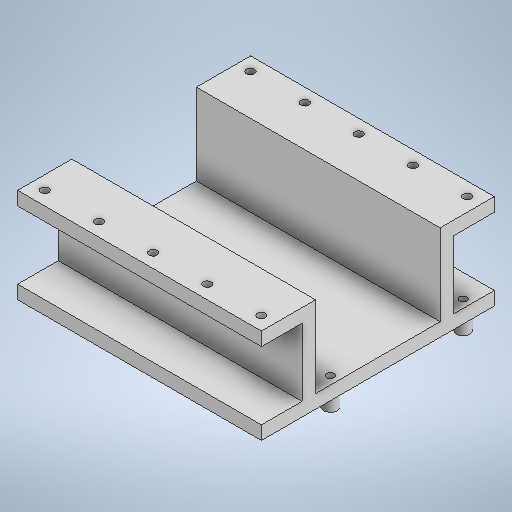
# Autodesk Inventor part: Battery_zig
Saved by Autodesk Inventor 2025 (Build 290162010, 162A)
## iProperties
Created: 2024-09-12
Part Number: Battery_zig
Material: Generic
Document SubType Name: Modeling
Designer: fist5
Density: 1 g/cm^3
Appearance: Default
Author: fist5
Autodesk Inventor part; units mm, degrees
ref_plane "YZ Plane" through (0, 0, 0) normal (1, 0, 0) x (0, 1, 0)
ref_plane "XZ Plane" through (0, 0, 0) normal (0, 1, 0) x (-1, 0, 0)
ref_plane "XY Plane" through (0, 0, 0) normal (0, 0, 1) x (1, 0, 0)
sketch "Sketch1" plane through (0, 0, 0) normal (0, 1, 0) x (-1, 0, 0)
  line L0 (45, -43) -> (-45, -43)
  line L1 (-45, -43) -> (-45, 43)
  line L2 (-45, 43) -> (45, 43)
  line L3 (45, 43) -> (45, -43)
  line L4 (45, -43) -> (-45, 43) construction
  line L5 (-45, -43) -> (45, 43) construction
  point P0 (0, 0)
  dimension "d0" = 90
  dimension "d1" = 86
  constraints: 12 end point, 2 midpoint, 2 parallel, 1 horizontal, 1 perpendicular
  measures "d0" distance between parallel lines of L1 L3
  measures "d1" distance between parallel lines of L2 L0
extrude "Extrusion1" add sketch "Sketch1" along normal blind 5
sketch "Sketch2" plane through (0, 5, 0) normal (0, 1, 0) x (1, 0, 0)
  line L0 (-45, 43) -> (-45, -43) projected
  line L1 (45, -43) -> (45, 43) projected
  line L2 (-45, 28) -> (45, 28)
  line L3 (45, 28) -> (45, 23)
  line L4 (45, 23) -> (-45, 23)
  line L5 (-45, 23) -> (-45, 28)
  line L6 (-45, -23) -> (45, -23)
  line L7 (45, -23) -> (45, -28)
  line L8 (45, -28) -> (-45, -28)
  line L9 (-45, -28) -> (-45, -23)
  point P0 (0, 0)
  point P1 (45, 0)
  point P2 (45, -28)
  point P3 (45, -23)
  point P4 (-45, 23)
  dimension "d4" = 46
  dimension "d5" = 23
  dimension "d6" = 5
  dimension "d7" = 5
  constraints: 16 end point, 4 parallel, 4 point on line, 2 horizontal, 2 perpendicular, 1 horizontal alignment, 1 midpoint
  measures "d4" distance between parallel lines of L6 L4
  measures "d5" distance of L3.end point (45, 0)
  measures "d6" distance between parallel lines of L4 L2
  measures "d7" distance between parallel lines of L8 L6
extrude "Extrusion2" add sketch "Sketch2" along normal blind 30 contours L2 L1 L4 L0 | L6 L1 L8 L0
sketch "Sketch3" plane through (45, 5, -28) normal (0, 0, -1) x (-1, 0, 0)
  line L0 (0, 0) -> (0, 30) projected
  line L1 (90, 0) -> (90, 30) projected
  line L2 (0, 30) -> (90, 30)
  line L3 (90, 30) -> (90, 25)
  line L4 (90, 25) -> (0, 25)
  line L5 (0, 25) -> (0, 30)
  point P0 (45, -5)
  point P1 (0, 25)
  dimension "d10" = 5
  constraints: 8 end point, 2 parallel, 1 horizontal, 1 perpendicular, 1 point on line
  measures "d10" distance between parallel lines of L2 L4
extrude "Extrusion3" add sketch "Sketch3" along normal blind 15
sketch "Sketch4" plane through (-45, 5, 28) normal (0, 0, 1) x (1, 0, 0)
  line L0 (90, 0) -> (90, 25) projected
  line L1 (0, 30) -> (90, 30)
  line L2 (90, 30) -> (90, 25)
  line L3 (90, 25) -> (0, 25)
  line L4 (0, 25) -> (0, 30)
  point P0 (45, -5)
  constraints: 8 end point, 2 parallel, 1 horizontal, 1 perpendicular
extrude "Extrusion4" add sketch "Sketch4" along normal blind 15
sketch "Sketch5" plane through (0, 35, 0) normal (0, 1, 0) x (1, 0, 0)
  circle A0 centre (40, 38) radius 1.5
  line L0 (-45, 43) -> (45, 43) projected
  line L1 (45, 23) -> (45, 43) projected
  circle A1 centre (40, -38) radius 1.5
  circle A2 centre (20, 38) radius 1.5
  circle A3 centre (20, -38) radius 1.5
  circle A4 centre (0, 38) radius 1.5
  circle A5 centre (0, -38) radius 1.5
  circle A6 centre (-20, 38) radius 1.5
  circle A7 centre (-20, -38) radius 1.5
  circle A8 centre (-40, 38) radius 1.5
  circle A9 centre (-40, -38) radius 1.5
  point P0 (0, 0)
  dimension "d15" = 3
  dimension "d21" = 5
  dimension "d22" = 5
  dimension "d25" = 76
  dimension "d28" = 20
  constraints: 10 centre point, 1 horizontal, 1 vertical, 18 other
  measures "d15" diameter of A0
  measures "d21" distance from line of L0 A0.centre
  measures "d22" distance from line of L1 A0.centre
  measures "d25" distance of A0.centre A1.centre
  measures "d28" distance of A0.centre A2.centre
extrude "Extrusion5" cut sketch "Sketch5" against normal up to surface (5 mm away)
sketch "Sketch8" plane through (0, 0, 0) normal (0, -1, 0) x (1, 0, 0)
  line L0 (42, 14.5) -> (-16, 14.5)
  line L1 (-16, 14.5) -> (-16, -34.5)
  line L2 (-16, -34.5) -> (42, -34.5)
  line L3 (42, -34.5) -> (42, 14.5)
  line L4 (42, 14.5) -> (-16, -34.5) construction
  line L5 (-16, 14.5) -> (42, -34.5) construction
  line L6 (45, 43) -> (45, -43) projected
  line L7 (-22.95, 17.94) -> (-42, 17.94)
  line L8 (-42, 17.94) -> (-42, -37.94)
  line L9 (-42, -37.94) -> (-22.95, -37.94)
  line L10 (-22.95, -37.94) -> (-22.95, 17.94)
  line L11 (-22.95, 17.94) -> (-42, -37.94) construction
  line L12 (-42, 17.94) -> (-22.95, -37.94) construction
  line L13 (-45, -43) -> (-45, 43) projected
  line L14 (45, 23) -> (45, -23) projected
  line L15 (45, -10) -> (-45, -10)
  circle A0 centre (42, 14.5) radius 1.35
  circle A1 centre (42, -34.5) radius 1.35
  circle A2 centre (-16, -34.5) radius 1.35
  circle A3 centre (-16, 14.5) radius 1.35
  circle A4 centre (-22.95, 17.94) radius 1.25
  circle A5 centre (-42, 17.94) radius 1.25
  circle A6 centre (-42, -37.94) radius 1.25
  circle A7 centre (-22.95, -37.94) radius 1.25
  point P0 (0, 0)
  point P1 (13, -10)
  point P2 (13, -34.5)
  point P3 (-32.475, -10)
  point P4 (-32.475, -37.94)
  dimension "d66" = 49
  dimension "d67" = 58
  dimension "d69" = 3
  dimension "d70" = 55.88
  dimension "d71" = 19.05
  dimension "d72" = 3
  dimension "d73" = 10
  dimension "d74" = 2.7
  dimension "d75" = 2.7
  dimension "d76" = 2.7
  dimension "d77" = 2.7
  dimension "d78" = 2.5
  dimension "d79" = 2.5
  dimension "d80" = 2.5
  dimension "d81" = 2.5
  constraints: 26 end point, 8 centre point, 8 coincident, 6 midpoint, 4 parallel, 3 perpendicular, 2 horizontal, 2 horizontal alignment, 2 point on line
  measures "d66" distance from line of point (13, -34.5) L0
  measures "d67" distance between parallel lines of L1 L3
  measures "d69" distance between parallel lines of L6 L3
  measures "d70" distance from line of point (-32.475, -37.94) L7
  measures "d71" distance between parallel lines of L8 L10
  measures "d72" distance between parallel lines of L13 L8
  measures "d73" distance from line of point (0, 0) L15
  measures "d74" diameter of A3
  measures "d75" diameter of A2
  measures "d76" diameter of A1
  measures "d77" diameter of A0
  measures "d78" diameter of A4
  measures "d79" diameter of A5
  measures "d80" diameter of A6
  measures "d81" diameter of A7
extrude "Extrusion8" cut sketch "Sketch8" against normal up to surface (5 mm away) contours A3 L1 L0 | L0 L1 A3 | A0 L3 L0 | L0 L3 A0 | A2 L2 L1 | L1 L2 A2 | A1 L2 L3 | L3 L2 A1 | A5 L8 L7 | L7 L8 A5 | A4 L10 L7 | L7 L10 A4 | A6 L9 L8 | L8 L9 A6 | A7 L9 L10 | L10 L9 A7
sketch "Sketch9" plane through (0, 0, 0) normal (0, -1, 0) x (1, 0, 0)
  line L0 (45, 28) -> (-45, 28) projected
  circle A0 centre (42, -34.5) radius 1.35 projected
  circle A1 centre (42, 14.5) radius 1.35 projected
  circle A2 centre (-22.95, -37.94) radius 1.25 projected
  circle A3 centre (-22.95, 17.94) radius 1.25 projected
  circle A4 centre (-16, -34.5) radius 1.35 projected
  circle A5 centre (-16, 14.5) radius 1.35 projected
  circle A6 centre (-42, -37.94) radius 1.25 projected
  circle A7 centre (-42, 17.94) radius 1.25 projected
  line L1 (-45, 43) -> (45, 43) projected
  line L2 (-45, -43) -> (-45, 43) projected
  line L3 (45, -43) -> (-45, -43) projected
  line L4 (45, 43) -> (45, -43) projected
  circle A8 centre (42, 14.5) radius 2.5
  circle A9 centre (42, -34.5) radius 2.5
  circle A10 centre (-16, -34.5) radius 2.5
  circle A11 centre (-22.95, -37.94) radius 2.5
  circle A12 centre (-42, -37.94) radius 2.5
  circle A13 centre (-42, 17.94) radius 2.5
  circle A14 centre (-22.95, 17.94) radius 2.5
  circle A15 centre (-16, 14.5) radius 2.5
  point P0 (0, 0)
  dimension "d84" = 5
  dimension "d85" = 5
  dimension "d86" = 5
  dimension "d87" = 5
  dimension "d88" = 5
  dimension "d89" = 5
  dimension "d90" = 5
  dimension "d91" = 5
  constraints: 8 centre point, 8 coincident
  measures "d84" diameter of A8
  measures "d85" diameter of A9
  measures "d86" diameter of A10
  measures "d87" diameter of A15
  measures "d88" diameter of A14
  measures "d89" diameter of A11
  measures "d90" diameter of A12
  measures "d91" diameter of A13
extrude "Extrusion9" add sketch "Sketch9" along normal blind 5 contours A0 | A8 | A9 | A10 | A11 | A12 | A13 | A14 | A15
body "Solid1"
